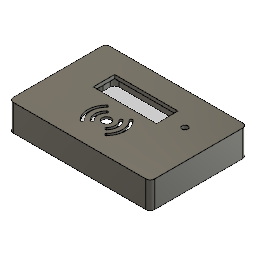
Gehäuse (Autodesk Fusion 360 design; units mm, degrees)
Autodesk Fusion 360 part; units mm, degrees
sketch "Skizze1" plane through (0, 0, 0) normal (0, 1, 0) x (1, 0, 0)
  line L0 (-79.5, 54.5) -> (79.5, 54.5)
  line L1 (79.5, 54.5) -> (79.5, -54.5)
  line L2 (79.5, -54.5) -> (-79.5, -54.5)
  line L3 (-79.5, -54.5) -> (-79.5, 54.5)
  line L4 (-79.5, 54.5) -> (79.5, -54.5) construction
  line L5 (79.5, 54.5) -> (-79.5, -54.5) construction
  dimension "d1" = 109
  dimension "d2" = 159
  constraint horizontal L0
  constraint perpendicular L0 L1
  constraint parallel L0 L2
  constraint parallel L1 L3
  constraint coincident L4 origin
  constraint coincident L5 origin
  measures "d1" distance of L0.end L1.end
  measures "d2" distance of L0.start L0.end
extrude "Extrusion1" add sketch "Skizze1" along normal blind 4
fillet "Abrundung1" radius 5 4 edges at (-79.5, 2, -54.5) (-79.5, 2, 54.5) (79.5, 2, 54.5) (79.5, 2, -54.5)
sketch "Skizze2" plane through (0, 4, 0) normal (0, 1, 0) x (-1, 0, 0)
  arc A0 (-79.5, -49.5) -> (-74.5, -54.5) centre (-74.5, -49.5) ccw
  line L0 (-74.5, -54.5) -> (74.5, -54.5)
  arc A1 (74.5, -54.5) -> (79.5, -49.5) centre (74.5, -49.5) ccw
  line L1 (79.5, -49.5) -> (79.5, 49.5)
  arc A2 (79.5, 49.5) -> (74.5, 54.5) centre (74.5, 49.5) ccw
  line L2 (74.5, 54.5) -> (-74.5, 54.5)
  arc A3 (-74.5, 54.5) -> (-79.5, 49.5) centre (-74.5, 49.5) ccw
  line L3 (-79.5, 49.5) -> (-79.5, -49.5)
  circle A4 centre (-46.5, -17.5) radius 3.25
  line L4 (44.5, -29.5) -> (-26.5, -29.5)
  line L5 (-26.5, -29.5) -> (-26.5, -5.5)
  line L6 (-26.5, -5.5) -> (44.5, -5.5)
  line L7 (44.5, -5.5) -> (44.5, -29.5)
  circle A5 centre (4.5, 19.5) radius 5
  line L8 (4.5, 19.5) -> (-9.2886, 5.7114) construction
  line L9 (4.5, 19.5) -> (-9.2886, 33.2886) construction
  arc A6 (-10.3492, 4.6508) -> (-8.2279, 6.7721) centre (-9.2886, 5.7114) ccw
  arc A7 (-8.2279, 32.2279) -> (-10.3492, 34.3492) centre (-9.2886, 33.2886) ccw
  arc A8 (-2.5711, 26.5711) -> (-4.6924, 28.6924) centre (-3.6317, 27.6317) ccw
  arc A9 (-4.6924, 10.3076) -> (-2.5711, 12.4289) centre (-3.6317, 11.3683) ccw
  arc A10 (-4.6924, 28.6924) -> (-4.6924, 10.3076) centre (4.5, 19.5) ccw
  arc A11 (-2.5711, 26.5711) -> (-2.5711, 12.4289) centre (4.5, 19.5) ccw
  arc A12 (-8.2279, 32.2279) -> (-8.2279, 6.7721) centre (4.5, 19.5) ccw
  arc A13 (-10.3492, 34.3492) -> (-10.3492, 4.6508) centre (4.5, 19.5) ccw
  line L10 (4.5, 19.5) -> (4.5, 4.5) construction
  arc A14 (19.3492, 34.3492) -> (17.2279, 32.2279) centre (18.2886, 33.2886) ccw
  arc A15 (17.2279, 6.7721) -> (19.3492, 4.6508) centre (18.2886, 5.7114) ccw
  arc A16 (19.3492, 4.6508) -> (19.3492, 34.3492) centre (4.5, 19.5) ccw
  arc A17 (11.5711, 12.4289) -> (13.6924, 10.3076) centre (12.6317, 11.3683) ccw
  arc A18 (11.5711, 12.4289) -> (11.5711, 26.5711) centre (4.5, 19.5) ccw
  arc A19 (13.6924, 28.6924) -> (11.5711, 26.5711) centre (12.6317, 27.6317) ccw
  arc A20 (17.2279, 6.7721) -> (17.2279, 32.2279) centre (4.5, 19.5) ccw
  arc A21 (13.6924, 10.3076) -> (13.6924, 28.6924) centre (4.5, 19.5) ccw
  point P0 (18.2886, 33.2886)
  point P1 (18.2886, 5.7114)
  dimension "d7" = 6.5
  dimension "d8" = 71
  dimension "d9" = 24
  dimension "d10" = 35
  dimension "d11" = 25
  dimension "d12" = 20
  dimension "d13" = 12
  dimension "d14" = 10
  dimension "d15" = 5
  dimension "d16" = 5
  dimension "d17" = 3
  dimension "d18" = 3
  dimension "d21" = 35
  dimension "d22" = 75
  dimension "d23" = 45
  constraint horizontal L4
  constraint vertical L5
  constraint horizontal L6
  constraint vertical L7
  constraint concentric A5 A11
  constraint concentric A10 A11
  constraint concentric A11 A12
  constraint concentric A10 A13
  constraint tangent A6 A13
  constraint tangent A6 A12
  constraint coincident A5.centre L8.start
  constraint coincident L8.end A6.centre
  constraint coincident L9.end A7.centre
  constraint coincident A9.centre L8
  constraint coincident A8.centre L9
  constraint tangent A7 A12
  constraint tangent A7 A13
  constraint tangent A9 A10
  constraint tangent A9 A11
  constraint tangent A8 A10
  constraint tangent A8 A11
  constraint vertical L10
  constraint symmetric L8.end L10 P1
  constraint symmetric L9.end L10 P0
  constraint symmetric A6.end L10 A15.start
  constraint symmetric A6.start L10 A15.end
  constraint symmetric A6 L10 A15
  constraint symmetric A7.end L10 A14.start
  constraint symmetric A7.start L10 A14.end
  constraint symmetric A7 L10 A14
  constraint symmetric A8.end L10 A19.start
  constraint symmetric A8.start L10 A18.end
  constraint symmetric A8 L10 A19
  constraint symmetric A9.end L10 A17.start
  constraint symmetric A9.start L10 A17.end
  constraint symmetric A9 L10 A17
  constraint symmetric A10 L10 A21
  constraint symmetric A11 L10 A18
  constraint symmetric A12 L10 A20
  constraint symmetric A13 L10 A16
  constraint perpendicular L8 L9
  measures "d7" diameter of A4
  measures "d8" distance of L4.start L4.end
  measures "d9" distance of L4.start L6.end
  measures "d10" distance of L1 L7
  measures "d11" distance of L0 L4
  measures "d12" distance of A4.centre L5
  measures "d13" distance of A4.centre L4
  measures "d14" diameter of A5
  measures "d15" distance of A5 A11
  measures "d16" distance of A10 A12
  measures "d17" distance of A10 A11
  measures "d18" distance of A12 A13
  measures "d21" distance of L2 A5.centre
  measures "d22" distance of L1 A5.centre
  measures "d23" angle of L8 L10
extrude "Extrusion2" cut sketch "Skizze2" against normal blind 4 contours A4 | L4 L5 L6 L7 | A5 | A6 A7 A12 A13 | A8 A9 A10 A11 | A14 A15 A16 A20 | A17 A18 A19 A21
sketch "Skizze3" plane through (0, 0, 0) normal (0, -1, 0) x (1, 0, 0)
  line L0 (26.5, -5.5) -> (26.5, -29.5)
  line L1 (26.5, -29.5) -> (-44.5, -29.5)
  line L2 (-44.5, -29.5) -> (-44.5, -5.5)
  line L3 (-44.5, -5.5) -> (26.5, -5.5)
  circle A0 centre (46.5, -17.5) radius 3.25
  arc A1 (74.5, -54.5) -> (79.5, -49.5) centre (74.5, -49.5) ccw
  line L4 (79.5, -49.5) -> (79.5, 49.5)
  arc A2 (79.5, 49.5) -> (74.5, 54.5) centre (74.5, 49.5) ccw
  line L5 (74.5, 54.5) -> (-74.5, 54.5)
  line L6 (-79.5, 49.5) -> (-79.5, -49.5)
  arc A3 (-79.5, -49.5) -> (-74.5, -54.5) centre (-74.5, -49.5) ccw
  line L7 (-74.5, -54.5) -> (74.5, -54.5)
sketch "Skizze4" plane through (0, 0, 0) normal (0, -1, 0) x (1, 0, 0)
  arc A0 (10.3492, 4.6508) -> (10.3492, 34.3492) centre (-4.5, 19.5) ccw
  arc A1 (8.2279, 6.7721) -> (10.3492, 4.6508) centre (9.2886, 5.7114) ccw
  arc A2 (8.2279, 6.7721) -> (8.2279, 32.2279) centre (-4.5, 19.5) ccw
  arc A3 (10.3492, 34.3492) -> (8.2279, 32.2279) centre (9.2886, 33.2886) ccw
  arc A4 (-17.2279, 32.2279) -> (-19.3492, 34.3492) centre (-18.2886, 33.2886) ccw
  arc A5 (-17.2279, 32.2279) -> (-17.2279, 6.7721) centre (-4.5, 19.5) ccw
  arc A6 (-19.3492, 4.6508) -> (-17.2279, 6.7721) centre (-18.2886, 5.7114) ccw
  arc A7 (-19.3492, 34.3492) -> (-19.3492, 4.6508) centre (-4.5, 19.5) ccw
  arc A8 (2.5711, 12.4289) -> (4.6924, 10.3076) centre (3.6317, 11.3683) ccw
  arc A9 (2.5711, 12.4289) -> (2.5711, 26.5711) centre (-4.5, 19.5) ccw
  arc A10 (4.6924, 28.6924) -> (2.5711, 26.5711) centre (3.6317, 27.6317) ccw
  arc A11 (4.6924, 10.3076) -> (4.6924, 28.6924) centre (-4.5, 19.5) ccw
  line L0 (26.5, -5.5) -> (26.5, -29.5)
  line L1 (26.5, -29.5) -> (-44.5, -29.5)
  line L2 (-44.5, -29.5) -> (-44.5, -5.5)
  line L3 (-44.5, -5.5) -> (26.5, -5.5)
  arc A12 (-13.6924, 28.6924) -> (-13.6924, 10.3076) centre (-4.5, 19.5) ccw
  arc A13 (-11.5711, 26.5711) -> (-13.6924, 28.6924) centre (-12.6317, 27.6317) ccw
  arc A14 (-11.5711, 26.5711) -> (-11.5711, 12.4289) centre (-4.5, 19.5) ccw
  arc A15 (-13.6924, 10.3076) -> (-11.5711, 12.4289) centre (-12.6317, 11.3683) ccw
  circle A16 centre (-4.5, 19.5) radius 5
  circle A17 centre (46.5, -17.5) radius 3.25
  arc A18 (74.5, -54.5) -> (79.5, -49.5) centre (74.5, -49.5) ccw
  line L4 (79.5, -49.5) -> (79.5, 49.5)
  arc A19 (79.5, 49.5) -> (74.5, 54.5) centre (74.5, 49.5) ccw
  line L5 (74.5, 54.5) -> (-74.5, 54.5)
  arc A20 (-74.5, 54.5) -> (-79.5, 49.5) centre (-74.5, 49.5) ccw
  line L6 (-79.5, 49.5) -> (-79.5, -49.5)
  arc A21 (-79.5, -49.5) -> (-74.5, -54.5) centre (-74.5, -49.5) ccw
  line L7 (-74.5, -54.5) -> (74.5, -54.5)
  line L8 (-29.75, 35.75) -> (20.75, 35.75)
  line L9 (20.75, 35.75) -> (20.75, 3.25)
  line L10 (20.75, 3.25) -> (-29.75, 3.25)
  line L11 (-29.75, 3.25) -> (-29.75, 35.75)
  line L12 (-29.75, 35.75) -> (20.75, 3.25) construction
  line L13 (20.75, 35.75) -> (-29.75, 3.25) construction
  point P0 (-4.5, 19.5)
  dimension "d50" = 50.5
  dimension "d51" = 32.5
  constraint horizontal L8
  constraint perpendicular L8 L9
  constraint parallel L8 L10
  constraint parallel L9 L11
  constraint coincident L12 P0
  constraint coincident L13 P0
  constraint coincident P0 A0.centre
  measures "d50" distance of L9.end L10.end
  measures "d51" distance of L8.end L9.end
extrude "Extrusion3" cut sketch "Skizze4" against normal blind 1.5 contours L8 L9 L10 L11
sketch "Skizze5" plane through (0, 0, 0) normal (0, -1, 0) x (1, 0, 0)
  line L0 (20.75, 35.75) -> (20.75, 3.25)
  line L1 (20.75, 3.25) -> (-29.75, 3.25)
  line L2 (-29.75, 3.25) -> (-29.75, 35.75)
  line L3 (-29.75, 35.75) -> (20.75, 35.75)
  line L4 (26.5, -5.5) -> (26.5, -29.5)
  line L5 (26.5, -29.5) -> (-44.5, -29.5)
  line L6 (-44.5, -29.5) -> (-44.5, -5.5)
  line L7 (-44.5, -5.5) -> (26.5, -5.5)
  circle A0 centre (46.5, -17.5) radius 3.25
  arc A1 (74.5, -54.5) -> (79.5, -49.5) centre (74.5, -49.5) ccw
  line L8 (79.5, -49.5) -> (79.5, 49.5)
  arc A2 (79.5, 49.5) -> (74.5, 54.5) centre (74.5, 49.5) ccw
  line L9 (74.5, 54.5) -> (-74.5, 54.5)
  arc A3 (-74.5, 54.5) -> (-79.5, 49.5) centre (-74.5, 49.5) ccw
  line L10 (-79.5, 49.5) -> (-79.5, -49.5)
  arc A4 (-79.5, -49.5) -> (-74.5, -54.5) centre (-74.5, -49.5) ccw
  line L11 (-74.5, -54.5) -> (74.5, -54.5)
  line L12 (74.5, 54.5) -> (-74.5, 54.5)
  arc A5 (-74.5, 54.5) -> (-79.5, 49.5) centre (-74.5, 49.5) ccw
  line L13 (-79.5, 49.5) -> (-79.5, -49.5)
  arc A6 (-79.5, -49.5) -> (-74.5, -54.5) centre (-74.5, -49.5) ccw
  line L14 (-74.5, -54.5) -> (74.5, -54.5)
  arc A7 (74.5, -54.5) -> (79.5, -49.5) centre (74.5, -49.5) ccw
  line L15 (79.5, -49.5) -> (79.5, 49.5)
  arc A8 (79.5, 49.5) -> (74.5, 54.5) centre (74.5, 49.5) ccw
  line L16 (-64.5, 49.5) -> (64.5, 49.5)
  line L17 (64.5, 49.5) -> (64.5, 31.5)
  line L18 (64.5, 31.5) -> (74.5, 31.5)
  line L19 (74.5, 31.5) -> (74.5, -31.5)
  line L20 (74.5, -31.5) -> (64.5, -31.5)
  line L21 (64.5, -31.5) -> (64.5, -49.5)
  line L22 (64.5, -49.5) -> (-64.5, -49.5)
  line L23 (-64.5, -49.5) -> (-64.5, -31.5)
  line L24 (-64.5, -31.5) -> (-74.5, -31.5)
  line L25 (-74.5, -31.5) -> (-74.5, 31.5)
  line L26 (-74.5, 31.5) -> (-64.5, 31.5)
  line L27 (-64.5, 31.5) -> (-64.5, 49.5)
  dimension "d54" = 5
  dimension "d55" = 5
  dimension "d56" = 5
  dimension "d57" = 5
  dimension "d58" = 15
  dimension "d59" = 23
  constraint parallel L9 L16
  constraint perpendicular L16 L17
  constraint perpendicular L17 L18
  constraint perpendicular L16 L19
  constraint perpendicular L19 L20
  constraint perpendicular L16 L21
  constraint perpendicular L19 L22
  constraint perpendicular L22 L23
  constraint perpendicular L19 L24
  constraint perpendicular L22 L25
  constraint perpendicular L25 L26
  constraint perpendicular L16 L27
  constraint equal L18 L26
  constraint equal L17 L27
  constraint equal L23 L27
  constraint equal L17 L21
  constraint equal L18 L20
  constraint equal L24 L26
  measures "d54" distance of L13 L25
  measures "d55" distance of L15 L19
  measures "d56" distance of L12 L16
  measures "d57" distance of L14 L22
  measures "d58" distance of L15 L17
  measures "d59" distance of L12 L18
extrude "Extrusion4" add sketch "Skizze5" along normal blind 26 contours A1 L8 A2 L9 A3 L10 A4 L11 L12 A5 L13 A6 L14 A7 L15 A8
fillet "Abrundung2" radius 5 12 edges at (64.5, -13, 49.5) (64.5, -13, 31.5) (74.5, -13, 31.5) (64.5, -13, -31.5) (74.5, -13, -31.5) (64.5, -13, -49.5) (-64.5, -13, -49.5) (-64.5, -13, -31.5) (-74.5, -13, -31.5) (-64.5, -13, 31.5) (-74.5, -13, 31.5) (-64.5, -13, 49.5)
equation "d13 = d9 / 2"
equation "d15 = d16"
equation "d17 = d18"
